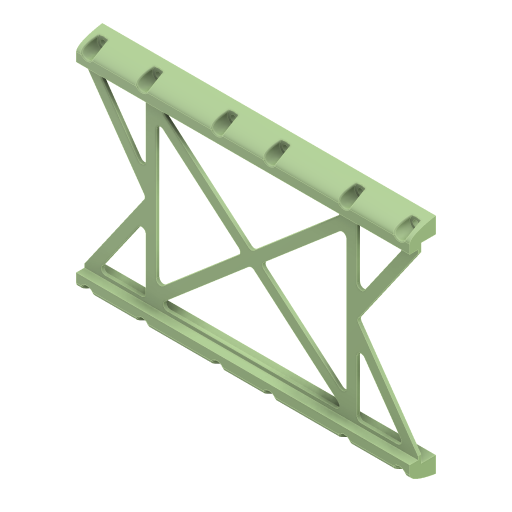
# Autodesk Inventor part: BodyStructure Centre Bottom
Saved by Autodesk Inventor 2023 (Build 270158000, 158)
## iProperties
Created: 2019-11-07
Part Number: BodyStructure Centre Bottom
Material: solidworks materials|ABS
Document SubType Name: Modeling
Designer: Jochen
Density: 1.02 g/cm^3
Appearance: 151,157,178
Sending System: SolidWorks 2017
Last Author: Felix
Last Saved: 2021-02-23
Author: Jochen
Autodesk Inventor part; units mm, degrees
note: some values were not read from the file. Chosen so that the rebuilt part matches the saved one: second side of "Extrusion1".
ref_plane "YZ Plane" through (0, 0, 0) normal (1, 0, 0) x (0, 1, 0)
ref_plane "XZ Plane" through (0, 0, 0) normal (0, 1, 0) x (-1, 0, 0)
ref_plane "Work Plane1" through (0, 0, 30) normal (0, 0, 1) x (1, 0, 0)
sketch "Sketch1" plane through (0, 0, 30) normal (0, 0, 1) x (1, 0, 0)
  line L0 (-80, -55) -> (80, -55)
  line L1 (80, 55) -> (-80, 55)
  line L2 (80, 42) -> (80, 42)
  line L3 (0, -77) -> (0, 77) construction
  line L4 (-112, 0) -> (112, 0) construction
  line L5 (-50.649, -42) -> (-50.649, -8.7287)
  line L6 (-45.649, 35.4185) -> (-45.649, -35.4185)
  line L7 (-50.649, -8.7287) -> (-73.9001, -42)
  line L8 (-80, -42) -> (-50.649, 0)
  line L9 (50.649, -8.7287) -> (73.9001, -42)
  line L10 (50.649, -42) -> (50.649, -8.7287)
  line L11 (45.649, 35.4185) -> (45.649, -35.4185)
  line L12 (80, -42) -> (50.649, 0)
  line L13 (50.649, 8.7287) -> (73.9001, 42)
  line L14 (80, 42) -> (50.649, 0)
  line L15 (50.649, 0) -> (50.649, 0)
  line L16 (50.649, 8.7287) -> (50.649, 42)
  line L17 (-50.649, 0) -> (-50.649, 0)
  line L18 (-80, 42) -> (-50.649, 0)
  line L19 (-50.649, 8.7287) -> (-73.9001, 42)
  line L20 (-80, 42) -> (-80, 42)
  line L21 (-50.649, 8.7287) -> (-50.649, 42)
  line L22 (73.9001, 42) -> (50.649, 42)
  line L23 (-73.9001, 42) -> (-50.649, 42)
  line L24 (-45.649, 42) -> (45.649, 42)
  line L25 (-80, -42) -> (-80, -42)
  line L26 (-50.649, -42) -> (-73.9001, -42)
  line L27 (45.649, -42) -> (-45.649, -42)
  line L28 (80, -42) -> (80, -42)
  line L29 (73.9001, -42) -> (50.649, -42)
  line L30 (80, -55) -> (80, -42)
  line L31 (80, 42) -> (80, 55)
  line L32 (-80, 55) -> (-80, 42)
  line L33 (-80, -42) -> (-80, -55)
  line L34 (-48.149, 55) -> (-48.149, -55) construction
  line L35 (-45.649, 42) -> (0, 2.9266)
  line L36 (0, 2.9266) -> (45.649, 42)
  line L37 (45.649, 35.4185) -> (4.2699, 0)
  line L38 (45.649, -35.4185) -> (4.2699, 0)
  line L39 (0, -2.9266) -> (45.649, -42)
  line L40 (-4.2699, 0) -> (-45.649, 35.4185)
  line L41 (-4.2699, 0) -> (-45.649, -35.4185)
  line L42 (0, -2.9266) -> (-45.649, -42)
  point P0 (0, 0)
  point P1 (-2.5, 42)
  point P2 (2.5, 42)
  point P3 (2.5, -42)
  point P4 (-2.5, -42)
  point P5 (50.649, 0)
  point P6 (-50.649, 0)
  dimension "d2" = 5
  dimension "d3" = 0
  dimension "d4" = 160
  dimension "d5" = 13
  dimension "d7" = 110
  dimension "d101" = 5
  dimension "d107" = 5
  constraints: 82 end point, 17 parallel, 15 collinear, 15 perpendicular, 11 point on line, 9 horizontal, 2 vertical, 19 other
  measures "d2" distance between parallel lines of L6 L5
  measures "d3" distance of L8.start L25.end
  measures "d4" distance of L0.start L0.end
  measures "d5" distance of L25.end L0.start
  measures "d7" distance between parallel lines of L1 L0
  measures "d101" distance between parallel lines of L8 L7
  measures "d107" distance between parallel lines of L42 L41
extrude "Extrusion1" add sketch "Sketch1" along normal blind 15.5
fillet "Fillet1" radius 2 22 edges at (-50.649, -42, 37.75) (-50.649, -8.7287, 37.75) (-73.9001, -42, 37.75) (-73.9001, 42, 37.75) (-50.649, 42, 37.75) (-50.649, 8.7287, 37.75) (50.649, -8.7287, 37.75) (50.649, -42, 37.75) (50.649, 42, 37.75) (50.649, 8.7287, 37.75) (73.9001, 42, 37.75) (73.9001, -42, 37.75) (-45.649, 35.4185, 37.75) (0, -2.9266, 37.75) (4.2699, 0, 37.75) (0, 2.9266, 37.75) (-4.2699, 0, 37.75) (-45.649, -35.4185, 37.75) (45.649, -35.4185, 37.75) (45.649, 35.4185, 37.75) (50.649, 0, 37.75) (-50.649, 0, 37.75)
fillet "Fillet1" radius 2 4 edges at (-45.649, 42, 37.75) (-45.649, -42, 37.75) (45.649, -42, 37.75) (45.649, 42, 37.75)
sketch "Sketch3" plane through (0, 0, 0) normal (1, 0, 0) x (0, 1, 0)
  line L0 (0, -9.1414) -> (0, 54.8485) construction
  line L1 (-78.4953, 0) -> (85.9718, 0) construction
  line L2 (-42, 45.5) -> (-55, 45.5) construction
  line L3 (-55, 45.5) -> (-42, 45.5) construction
  line L4 (-42, 45.5) -> (-1.1456, 45.5) construction
  line L5 (1.1456, 45.5) -> (42, 45.5) construction
  line L6 (42, 45.5) -> (55, 45.5) construction
  line L7 (55, 45.5) -> (42, 45.5) construction
  line L8 (42, 45.5) -> (1.1456, 45.5) construction
  line L9 (-1.1456, 45.5) -> (-42, 45.5) construction
  line L10 (13.9365, 45.5) -> (38.8544, 45.5) construction
  line L11 (42, 45.5) -> (38.8544, 45.5) construction
  line L12 (40, 45.5) -> (42, 45.5) construction
  line L13 (40, 45.5) -> (15.0821, 45.5) construction
  line L14 (13.9365, 45.5) -> (15.0821, 45.5) construction
  line L15 (15.0821, 45.5) -> (40, 45.5) construction
  line L16 (42, 45.5) -> (40, 45.5) construction
  line L17 (38.8544, 45.5) -> (42, 45.5) construction
  line L18 (38.8544, 45.5) -> (13.9365, 45.5) construction
  line L19 (15.0821, 45.5) -> (13.9365, 45.5) construction
  line L20 (-13.9365, 45.5) -> (-38.8544, 45.5) construction
  line L21 (-40, 45.5) -> (-42, 45.5) construction
  line L22 (-40, 45.5) -> (-15.0821, 45.5) construction
  line L23 (-13.9365, 45.5) -> (-15.0821, 45.5) construction
  line L24 (-38.8544, 45.5) -> (-42, 45.5) construction
  line L25 (-38.8544, 45.5) -> (-13.9365, 45.5) construction
  line L26 (-15.0821, 45.5) -> (-13.9365, 45.5) construction
  line L27 (-15.0821, 45.5) -> (-40, 45.5) construction
  line L28 (-42, 45.5) -> (-40, 45.5) construction
  line L29 (-42, 30) -> (-55, 30) construction
  line L30 (-1.1456, 30) -> (-42, 30) construction
  line L31 (42, 30) -> (1.1456, 30) construction
  line L32 (55, 30) -> (42, 30) construction
  line L33 (42, 30) -> (55, 30) construction
  line L34 (1.1456, 30) -> (42, 30) construction
  line L35 (-42, 30) -> (-1.1456, 30) construction
  line L36 (-55, 30) -> (-42, 30) construction
  line L37 (15.0821, 30) -> (13.9365, 30) construction
  line L38 (40, 30) -> (15.0821, 30) construction
  line L39 (42, 30) -> (40, 30) construction
  line L40 (38.8544, 30) -> (42, 30) construction
  line L41 (13.9365, 30) -> (38.8544, 30) construction
  line L42 (13.9365, 30) -> (15.0821, 30) construction
  line L43 (38.8544, 30) -> (13.9365, 30) construction
  line L44 (42, 30) -> (38.8544, 30) construction
  line L45 (40, 30) -> (42, 30) construction
  line L46 (15.0821, 30) -> (40, 30) construction
  line L47 (-15.0821, 30) -> (-13.9365, 30) construction
  line L48 (-40, 30) -> (-15.0821, 30) construction
  line L49 (-42, 30) -> (-40, 30) construction
  line L50 (-13.9365, 30) -> (-38.8544, 30) construction
  line L51 (-40, 30) -> (-42, 30) construction
  line L52 (-15.0821, 30) -> (-40, 30) construction
  line L53 (-13.9365, 30) -> (-15.0821, 30) construction
  line L54 (-38.8544, 30) -> (-13.9365, 30) construction
  line L55 (-42, 30) -> (-38.8544, 30) construction
  line L56 (55, 30) -> (55, 45.5) construction
  line L57 (55, 30) -> (55, 45.5) construction
  line L58 (-55, 30) -> (-55, 45.5) construction
  line L59 (-55, 30) -> (-55, 45.5) construction
  line L60 (-37, 30) -> (-37, 45.5) construction
  line L61 (-37, 30) -> (-37, 45.5) construction
  line L62 (-55, 30) -> (-55, 45.5)
  line L63 (-47.5, 45.5) -> (-45, 45.5)
  line L64 (-43.75, 41.5) -> (43.75, 41.5)
  line L65 (55, 45.5) -> (55, 30)
  line L66 (55, 30) -> (-55, 30)
  line L67 (-46.25, 45.5) -> (-46.25, 30) construction
  line L68 (-38.8544, 30) -> (-42, 30) projected
  line L69 (-42, 45.5) -> (-38.8544, 45.5) projected
  line L70 (42, 45.5) -> (42, 30) projected
  line L71 (42, 30) -> (42, 45.5) projected
  line L72 (1.1456, 30) -> (-1.1456, 30) projected
  line L73 (-1.1456, 30) -> (1.1456, 30) projected
  line L74 (1.1456, 45.5) -> (-1.1456, 45.5) projected
  line L75 (-1.1456, 45.5) -> (1.1456, 45.5) projected
  line L76 (-43.75, 41.5) -> (-43.75, 45.5)
  line L77 (-43.75, 45.5) -> (-45, 45.5)
  line L78 (-55, 45.5) -> (-42, 45.5) projected
  line L79 (-47.5, 45.5) -> (-55, 45.5)
  line L80 (-55, 30) -> (-55, 45.5) projected
  line L81 (42, 45.5) -> (55, 45.5) projected
  line L82 (43.75, 41.5) -> (43.75, 45.5)
  line L83 (55, 45.5) -> (43.75, 45.5)
  point P0 (0, 0)
  point P1 (-55, 39.9819)
  point P2 (62.4765, 45.5)
  dimension "d114" = 4
  dimension "d115" = 87.5
  constraints: 25 end point, 8 point on line, 4 perpendicular, 3 collinear, 2 horizontal, 2 vertical, 1 midpoint, 1 parallel, 6 other
  measures "d114" distance of L64.start L76.end
  measures "d115" distance between parallel lines of L76 L82
extrude "Extrusion3" cut sketch "Sketch3" along normal through all both and the other way through all contours L62 L78 L63 L77 L76 L64 L70 L66 | L70 L64 L82 L81 L65 L66 keep common part
sketch "Sketch12" plane through (80, -55, 30) normal (1, 0, 0) x (0, 0, -1)
  line L0 (0, 13) -> (0, 0) projected
  line L1 (0, 0) -> (-15.5, 0) projected
  line L2 (-15.5, 110) -> (0, 110) projected
  line L3 (0, 110) -> (0, 97) projected
  line L4 (-11.5, 13) -> (0, 13) projected
  line L5 (0, 97) -> (-11.5, 97) projected
  line L6 (-11.5, 97) -> (-11.5, 98.75) projected
  line L7 (-11.5, 98.75) -> (-15.5, 98.75) projected
  line L8 (-15.5, 98.75) -> (-15.5, 110) projected
  line L9 (-15.5, 0) -> (-15.5, 11.25) projected
  line L10 (-15.5, 11.25) -> (-11.5, 11.25) projected
  line L11 (-11.5, 11.25) -> (-11.5, 13) projected
  point P0 (30, 55)
  point P1 (-11.5, 11.4559)
  point P2 (-11.5, 98.5441)
sketch "Sketch15" plane through (0, 0, 0) normal (0, 1, 0) x (-1, 0, 0)
  line L0 (-51.089, 41.5) -> (-45.649, 41.5) construction
  line L1 (-45.649, 41.5) -> (-45.649, 30) construction
  line L2 (-45.649, 30) -> (-51.089, 30) construction
  line L3 (-51.089, 30) -> (-51.089, 41.5) construction
  line L4 (-5.3456, 41.5) -> (5.3456, 41.5) construction
  line L5 (5.3456, 41.5) -> (5.3456, 30) construction
  line L6 (5.3456, 30) -> (-5.3456, 30) construction
  line L7 (-5.3456, 30) -> (-5.3456, 41.5) construction
  line L8 (45.649, 41.5) -> (51.089, 41.5) construction
  line L9 (51.089, 41.5) -> (51.089, 30) construction
  line L10 (51.089, 30) -> (45.649, 30) construction
  line L11 (45.649, 30) -> (45.649, 41.5) construction
  line L12 (-27.5, 45.5) -> (-8.5, 45.5)
  line L13 (-8.5, 44.5) -> (-8.5, 30)
  line L14 (-8.5, 30) -> (-28.5, 30)
  line L15 (-28.5, 30) -> (-28.5, 44.5)
  line L16 (-8.5, 30) -> (8.5, 30)
  line L17 (8.5, 30) -> (8.5, 44.5)
  line L18 (7.5, 45.5) -> (-7.5, 45.5)
  line L19 (-8.5, 45.5) -> (-8.5, 30)
  line L20 (8.5, 30) -> (28.5, 30)
  line L21 (28.5, 30) -> (28.5, 44.5)
  line L22 (27.5, 45.5) -> (8.5, 45.5)
  line L23 (8.5, 45.5) -> (8.5, 30)
  line L24 (80, 45.5) -> (-80, 45.5) construction
  line L25 (-42.3485, 30) -> (-6.0451, 30) construction
  arc A0 (-27.5, 45.5) -> (-28.5, 44.5) centre (-27.5, 44.5) ccw
  arc A1 (28.5, 44.5) -> (27.5, 45.5) centre (27.5, 44.5) ccw
  arc A2 (8.5, 44.5) -> (7.5, 45.5) centre (7.5, 44.5) ccw
  arc A3 (-7.5, 45.5) -> (-8.5, 44.5) centre (-7.5, 44.5) ccw
  line L26 (-8.5, 45.5) -> (-7.5, 45.5)
  line L27 (7.5, 45.5) -> (8.5, 45.5)
  line L28 (28.5, 36.2) -> (-28.5, 36.2)
  point P0 (0, 0)
  point P1 (-28.5, 45.5)
  point P2 (28.5, 45.5)
  point P3 (28.5, 37.25)
  point P4 (-8.5, 36.2)
  point P5 (8.5, 36.2)
  dimension "d123" = 37
  dimension "d124" = 37
  dimension "d125" = 51.5
  dimension "d126" = 51.5
  dimension "d131" = 1
  dimension "d133" = 9.3
  constraints: 30 end point, 16 point on line, 10 tangent, 9 point on circle, 6 parallel, 4 centre point, 4 horizontal, 3 equal radius, 3 perpendicular, 2 collinear, 1 midpoint
  measures "d123" distance between parallel lines of L17 L15
  measures "d124" distance from line of point (28.5, 37.25) L13
  measures "d125" distance from line of L15 L24.end
  measures "d126" horizontal distance of L24.start L20.end
  measures "d131" radius of A0
  measures "d133" distance between parallel lines of L28 L24
sketch "Sketch16" plane through (0, 0, 0) normal (1, 0, 0) x (0, 1, 0)
  line L0 (-80.8624, 0) -> (80.8624, 0) construction
  line L1 (-80.8624, 0) -> (80.8624, 0) construction
  line L2 (0, -29.7721) -> (0, 58.7721) construction
  line L3 (-48, 45.5) -> (-48, -16.5) construction
  line L4 (55, 45.5) -> (43.75, 45.5) construction
  line L5 (48, 45.5) -> (48, -16.5) construction
  line L6 (-43.75, 45.5) -> (-55, 45.5) construction
  ellipse E0 centre (-48, 14.5) end of major axis (-48, 45.5) minor radius 7 (-48, 45.5) -> (-55, 14.5) ccw
  line L7 (-55, 30) -> (-55, 45.5) projected
  line L8 (-55, 30) -> (-55, 14.5) construction
  line L9 (-48, 45.5) -> (-55, 45.5)
  line L10 (-55, 45.5) -> (-55, 14.5)
  ellipse E1 centre (48, 14.5) end of major axis (48, 45.5) minor radius 7 (48, -16.5) -> (55, 14.5) ccw construction
  line L11 (48, 45.5) -> (55, 45.5)
  line L12 (55, 45.5) -> (55, 14.5)
  ellipse E2 centre (-48, 14.5) end of major axis (-48, 45.5) minor radius 7 (-55, 14.5) -> (-48, -16.5) ccw construction
  ellipse E3 centre (48, 14.5) end of major axis (48, 45.5) minor radius 7 (55, 14.5) -> (48, 45.5) ccw
  line L13 (55, 14.5) -> (-55, 14.5) construction
  point P0 (0, 0)
  dimension "d138" = 62
  dimension "d139" = 7
  constraints: 16 end point, 8 vertical, 2 collinear, 2 midpoint, 2 point on line, 1 horizontal, 1 parallel, 17 other
  measures "d138" distance of L3.end L3.start
  measures "d139" distance from line of L3 L6.end
extrude "Extrusion16" cut sketch "Sketch16" along normal through all both and the other way through all
sketch "Sketch5" plane through (0, 0, 0) normal (0, 1, 0) x (-1, 0, 0)
  line L0 (112, 0) -> (-112, 0) construction
  line L1 (0, -9.1414) -> (0, 54.8485) construction
  line L2 (80, 41.5) -> (80, 45.5) construction
  line L3 (-80, 30) -> (-80, 45.5) construction
  line L4 (-80, 30) -> (80, 30) construction
  line L5 (80, 30) -> (80, 45.5) construction
  line L6 (80, 39.5) -> (80, 41.5) construction
  line L7 (-80, 41.5) -> (-80, 39.5) construction
  line L8 (-52, 34.5) -> (-52, 33)
  line L9 (-52, 33) -> (-45, 33)
  line L10 (-45, 33) -> (-45, 40)
  line L11 (-45, 40) -> (-16, 40)
  line L12 (-16, 40) -> (-16, 33)
  line L13 (-16, 33) -> (-9, 33)
  line L14 (-9, 33) -> (-9, 40)
  line L15 (-9, 40) -> (9, 40)
  line L16 (9, 40) -> (9, 33)
  line L17 (9, 33) -> (16, 33)
  line L18 (16, 33) -> (16, 40)
  line L19 (16, 40) -> (45, 40)
  line L20 (45, 40) -> (45, 33)
  line L21 (45, 33) -> (52, 33)
  line L22 (52, 33) -> (52, 34.5)
  line L23 (80, 34.5) -> (80, 45.5)
  line L24 (80, 30) -> (-80, 30) construction
  line L25 (-80, 45.5) -> (-80, 34.5)
  line L26 (80, 41.5) -> (-80, 41.5)
  line L27 (52, 34.5) -> (80, 34.5)
  line L28 (-80, 34.5) -> (-52, 34.5)
  line L29 (52, 40) -> (45, 40) construction
  line L30 (80, 45.5) -> (-80, 45.5) projected
  line L31 (-80, 45.5) -> (80, 45.5)
  line L32 (-80, 45.5) -> (80, 45.5) projected
  line L33 (-52.649, 30) -> (-52.649, 41.5) projected
  line L34 (53, 34.5) -> (53, 33)
  line L35 (53, 33) -> (52, 33)
  line L36 (-53, 34.5) -> (-53, 33)
  line L37 (-53, 33) -> (-52, 33)
  line L38 (-45, 33) -> (45, 33)
  line L39 (45.649, 41.5) -> (45.649, 30) projected
  line L40 (53, 33) -> (80, 33)
  line L41 (-53, 33) -> (-80, 33)
  line L42 (-80, 34.5) -> (-80, 33)
  line L43 (-80, 30) -> (-80, 41.5) projected
  line L44 (80, 34.5) -> (80, 33)
  line L45 (80, 30) -> (80, 41.5) projected
  point P0 (0, 0)
  point P1 (61.4737, 40)
  point P2 (56.7369, 40)
  point P3 (48.5, 33)
  point P4 (-52.649, 34.5)
  dimension "d47" = 7
  dimension "d48" = 9
  dimension "d51" = 11
  dimension "d96" = 7
  dimension "d102" = 48.5
  dimension "d118" = 12.5
  dimension "d145" = 27
  dimension "d146" = 27
  constraints: 62 end point, 16 point on line, 15 perpendicular, 6 collinear, 3 vertical, 1 horizontal, 1 midpoint, 1 parallel, 2 other
  measures "d47" distance between parallel lines of L22 L20
  measures "d48" distance between parallel lines of L1 L16
  measures "d51" distance from line of L2.end L27
  measures "d96" distance between parallel lines of L21 L29
  measures "d102" distance from line of L1 point (48.5, 33)
  measures "d118" distance between parallel lines of L30 L13
  measures "d145" distance between parallel lines of L5 L34
  measures "d146" distance between parallel lines of L3 L36
extrude "Extrusion5" cut sketch "Sketch5" along normal through all both and the other way through all keep common part
sketch "Sketch6" plane through (0, 0, 0) normal (1, 0, 0) x (0, 1, 0)
  line L0 (0, -9.1414) -> (0, 54.8485) construction
  line L1 (-77, 0) -> (77, 0) construction
  line L2 (-38.535, 41.5) -> (-36.9915, 41.5) construction
  line L3 (-45.875, 40) -> (-45.875, 25)
  line L4 (-45.875, 25) -> (45.875, 25)
  line L5 (45.875, 25) -> (45.875, 40)
  line L6 (-45.875, 40) -> (45.875, 40)
  line L7 (42, 40) -> (51.9805, 40) projected
  line L8 (-43.75, 45.5) -> (-48, 45.5) construction
  line L9 (45.875, 25) -> (53.125, 25)
  line L10 (53.125, 25) -> (53.125, 40)
  line L11 (45.875, 40) -> (53.125, 40)
  line L12 (-45.875, 40) -> (-53.125, 40)
  line L13 (-53.125, 40) -> (-53.125, 25)
  line L14 (-53.125, 25) -> (-45.875, 25)
  line L15 (55, 33) -> (55, 40) projected
  line L16 (55, 33) -> (55, 25)
  line L17 (55, 25) -> (53.125, 25)
  line L18 (55, 33) -> (55, 40)
  line L19 (55, 40) -> (53.125, 40)
  line L20 (-53.125, 25) -> (-55, 25)
  line L21 (-55, 25) -> (-55, 40)
  line L22 (-55, 40) -> (-53.125, 40)
  point P0 (0, 0)
  point P1 (-45.875, 32.5)
  point P2 (54.9365, 40)
  point P3 (-45, 45.5)
  point P4 (-47.5, 45.5)
  point P5 (-45.875, 45.5)
  point P6 (55, 39.5)
  point P7 (-55, 33)
  point P8 (55, 39.5)
  point P9 (54.9365, 40)
  point P10 (-54.9365, 40)
  point P11 (-54.9161, 45.5)
  point P12 (-50, 45.5)
  point P13 (54.9791, 40)
  point P14 (-42, 45.5)
  point P15 (-55, 45.5)
  dimension "d75" = 1.5
  dimension "d104" = 15
  dimension "d106" = 7.25
  constraints: 37 end point, 6 perpendicular, 6 point on line, 4 collinear, 2 horizontal, 2 vertical, 1 midpoint, 1 parallel, 3 other
  measures "d75" distance between parallel lines of L6 L2
  measures "d104" distance from line of L6 L3.end
  measures "d106" distance between parallel lines of L5 L10
extrude "Extrusion6" cut sketch "Sketch6" along normal mid plane 160 contours L6 L5 L4 L3
sketch "Sketch9" plane through (45, -54.9365, 40) normal (0, 0, -1) x (-1, 0, 0)
  line L0 (-35, 100.8115) -> (-35, 106.917) projected
  line L1 (-35, 2.956) -> (-35, 9.0615) projected
  line L2 (125, 106.917) -> (125, 100.8115) projected
  line L3 (125, 9.0615) -> (125, 2.956) projected
  circle A0 centre (-30, 104.9365) radius 1.5
  circle A1 centre (32.5, 104.9365) radius 1.5
  circle A2 centre (-3.5, 104.9365) radius 1.5
  circle A3 centre (57.5, 104.9365) radius 1.5
  circle A4 centre (93.5, 104.9365) radius 1.5
  circle A5 centre (120, 104.9365) radius 1.5
  circle A6 centre (120, 4.9365) radius 1.5
  circle A7 centre (93.5, 4.9365) radius 1.5
  circle A8 centre (57.5, 4.9365) radius 1.5
  circle A9 centre (-3.5, 4.9365) radius 1.5
  circle A10 centre (32.5, 4.9365) radius 1.5
  circle A11 centre (-30, 4.9365) radius 1.5
  line L4 (-30, 104.9365) -> (120, 104.9365) construction
  line L5 (120, 104.9365) -> (120, 4.9365) construction
  line L6 (120, 4.9365) -> (-30, 4.9365) construction
  line L7 (-30, 4.9365) -> (-30, 104.9365) construction
  line L8 (157, 54.9365) -> (-67, 54.9365) construction
  line L9 (45, -22.0635) -> (45, 131.9365) construction
  line L10 (32.5, 104.9365) -> (32.5, 4.9365) construction
  line L11 (-3.5, 4.9365) -> (-3.5, 104.9365) construction
  line L12 (93.5, 104.9365) -> (93.5, 4.9365) construction
  line L13 (57.5, 104.9365) -> (57.5, 4.9365) construction
  circle A12 centre (-30, 4.9365) radius 2.9
  circle A13 centre (-3.5, 4.9365) radius 2.9
  circle A14 centre (32.5, 4.9365) radius 2.9
  circle A15 centre (57.5, 4.9365) radius 2.9
  circle A16 centre (93.5, 4.9365) radius 2.9
  circle A17 centre (120, 4.9365) radius 2.9
  circle A18 centre (120, 104.9365) radius 2.9
  circle A19 centre (93.5, 104.9365) radius 2.9
  circle A20 centre (57.5, 104.9365) radius 2.9
  circle A21 centre (32.5, 104.9365) radius 2.9
  circle A22 centre (-3.5, 104.9365) radius 2.9
  circle A23 centre (-30, 104.9365) radius 2.9
  line L14 (125, 108.4365) -> (-35, 108.4365)
  line L15 (-35, 1.4365) -> (125, 1.4365)
  line L16 (-35, 9.0615) -> (125, 9.0615) projected
  line L17 (125, 100.8115) -> (-35, 100.8115) projected
  line L18 (97.7, 1.4365) -> (97.7, -0.0635)
  line L19 (97.7, 108.4365) -> (97.7, 109.9365)
  line L20 (125, -0.0635) -> (-35, -0.0635) projected
  line L21 (-7.7, -0.0635) -> (-7.7, 1.4365)
  line L22 (-7.7, 108.4365) -> (-7.7, 109.9365)
  line L23 (125, 109.9365) -> (-35, 109.9365) projected
  line L24 (125, 2.956) -> (-35, 2.956) projected
  line L25 (-35, 106.917) -> (125, 106.917) projected
  arc A24 (-25.0624, 96.9365) -> (-26.7018, 93.7909) centre (-25.0624, 94.9365) ccw projected
  line L26 (-26.7018, 93.7909) -> (-9.2884, 68.873) projected
  arc A25 (-9.2884, 68.873) -> (-5.649, 70.0186) centre (-7.649, 70.0186) ccw projected
  line L27 (-5.649, 70.0186) -> (-5.649, 94.9365) projected
  arc A26 (-5.649, 94.9365) -> (-7.649, 96.9365) centre (-7.649, 94.9365) ccw projected
  line L28 (-7.649, 96.9365) -> (-25.0624, 96.9365) projected
  line L29 (99.2884, 68.873) -> (116.7018, 93.7909) projected
  arc A27 (116.7018, 93.7909) -> (115.0624, 96.9365) centre (115.0624, 94.9365) ccw projected
  line L30 (115.0624, 96.9365) -> (97.649, 96.9365) projected
  arc A28 (97.649, 96.9365) -> (95.649, 94.9365) centre (97.649, 94.9365) ccw projected
  line L31 (95.649, 94.9365) -> (95.649, 70.0186) projected
  arc A29 (95.649, 70.0186) -> (99.2884, 68.873) centre (97.649, 70.0186) ccw projected
  arc A30 (99.2884, 41) -> (95.649, 39.8543) centre (97.649, 39.8543) ccw projected
  line L32 (95.649, 39.8543) -> (95.649, 14.9365) projected
  arc A31 (95.649, 14.9365) -> (97.649, 12.9365) centre (97.649, 14.9365) ccw projected
  line L33 (97.649, 12.9365) -> (115.0624, 12.9365) projected
  arc A32 (115.0624, 12.9365) -> (116.7018, 16.0821) centre (115.0624, 14.9365) ccw projected
  line L34 (116.7018, 16.0821) -> (99.2884, 41) projected
  line L35 (86.5373, 16.4559) -> (46.3005, 50.8966) projected
  arc A33 (46.3005, 50.8966) -> (43.6995, 50.8966) centre (45, 49.3772) ccw projected
  line L36 (43.6995, 50.8966) -> (3.4627, 16.4559) projected
  arc A34 (3.4627, 16.4559) -> (4.7632, 12.9365) centre (4.7632, 14.9365) ccw projected
  line L37 (4.7632, 12.9365) -> (85.2368, 12.9365) projected
  arc A35 (85.2368, 12.9365) -> (86.5373, 16.4559) centre (85.2368, 14.9365) ccw projected
  line L38 (3.4627, 93.4171) -> (43.6995, 58.9763) projected
  arc A36 (43.6995, 58.9763) -> (46.3005, 58.9763) centre (45, 60.4957) ccw projected
  line L39 (46.3005, 58.9763) -> (86.5373, 93.4171) projected
  arc A37 (86.5373, 93.4171) -> (85.2368, 96.9365) centre (85.2368, 94.9365) ccw projected
  line L40 (85.2368, 96.9365) -> (4.7632, 96.9365) projected
  arc A38 (4.7632, 96.9365) -> (3.4627, 93.4171) centre (4.7632, 94.9365) ccw projected
  line L41 (2.6515, 22.3431) -> (38.9549, 53.4171) projected
  arc A39 (38.9549, 53.4171) -> (38.9549, 56.4559) centre (37.6544, 54.9365) ccw projected
  line L42 (38.9549, 56.4559) -> (2.6515, 87.5299) projected
  arc A40 (2.6515, 87.5299) -> (-0.649, 86.0105) centre (1.351, 86.0105) ccw projected
  line L43 (-0.649, 86.0105) -> (-0.649, 23.8625) projected
  arc A41 (-0.649, 23.8625) -> (2.6515, 22.3431) centre (1.351, 23.8625) ccw projected
  line L44 (90.649, 23.8625) -> (90.649, 86.0105) projected
  arc A42 (90.649, 86.0105) -> (87.3485, 87.5299) centre (88.649, 86.0105) ccw projected
  line L45 (87.3485, 87.5299) -> (51.0451, 56.4559) projected
  arc A43 (51.0451, 56.4559) -> (51.0451, 53.4171) centre (52.3456, 54.9365) ccw projected
  line L46 (51.0451, 53.4171) -> (87.3485, 22.3431) projected
  arc A44 (87.3485, 22.3431) -> (90.649, 23.8625) centre (88.649, 23.8625) ccw projected
  line L47 (-5.649, 14.9365) -> (-5.649, 39.8543) projected
  arc A45 (-5.649, 39.8543) -> (-9.2884, 41) centre (-7.649, 39.8543) ccw projected
  line L48 (-9.2884, 41) -> (-26.7018, 16.0821) projected
  arc A46 (-26.7018, 16.0821) -> (-25.0624, 12.9365) centre (-25.0624, 14.9365) ccw projected
  line L49 (-25.0624, 12.9365) -> (-7.649, 12.9365) projected
  arc A47 (-7.649, 12.9365) -> (-5.649, 14.9365) centre (-7.649, 14.9365) ccw projected
  line L50 (125, 96.9365) -> (96.4496, 56.0821) projected
  arc A48 (96.4496, 56.0821) -> (96.4496, 53.7909) centre (98.089, 54.9365) ccw projected
  line L51 (96.4496, 53.7909) -> (125, 12.9365) projected
  line L52 (125, 12.9365) -> (125, 9.0615) projected
  line L53 (125, 100.8115) -> (125, 96.9365) projected
  line L54 (-35, 9.0615) -> (-35, 12.9365) projected
  line L55 (-35, 12.9365) -> (-6.4496, 53.7909) projected
  arc A49 (-6.4496, 53.7909) -> (-6.4496, 56.0821) centre (-8.089, 54.9365) ccw projected
  line L56 (-6.4496, 56.0821) -> (-35, 96.9365) projected
  line L57 (-35, 96.9365) -> (-35, 100.8115) projected
  point P0 (45, 54.9365)
  point P1 (42.5, 12.9365)
  point P2 (-6, 80.6486)
  point P3 (-6, 19.2244)
  point P4 (-6, 14.9365)
  point P5 (47.5, 86.9365)
  point P6 (42.5, 76.9365)
  point P7 (42.5, 22.9365)
  point P8 (47.5, 76.9365)
  point P9 (47.5, 22.9365)
  point P10 (-6, 36.0374)
  point P11 (98.4175, 46.8521)
  point P12 (45, 52.0098)
  point P13 (45, 57.8631)
  point P14 (-5.649, 54.9365)
  point P15 (95.649, 54.9365)
  point P16 (0, 109.9365)
  point P17 (36, -0.0635)
  point P18 (29, -0.0635)
  point P19 (0, -0.0635)
  point P20 (1, 109.9365)
  point P21 (28, 109.9365)
  point P22 (37, 109.9365)
  point P23 (53, 109.9365)
  point P24 (62, 109.9365)
  point P25 (89, 109.9365)
  point P26 (98, 109.9365)
  point P27 (89, -0.0635)
  point P28 (62, -0.0635)
  point P29 (53, -0.0635)
  point P30 (37, -0.0635)
  point P31 (28, -0.0635)
  point P32 (1, -0.0635)
  point P33 (-8, -0.0635)
  point P34 (0, 101.8115)
  point P35 (90, 101.8115)
  point P36 (90, 8.0615)
  point P37 (0, 8.0615)
  point P38 (36.5, -0.0635)
  point P39 (16.5, 109.9365)
  point P40 (16.5, -0.0635)
  dimension "d61" = 3
  dimension "d63" = 100
  dimension "d64" = 75
  dimension "d65" = 48.5
  dimension "d66" = 12.5
  dimension "d69" = 5.8
  constraints: 28 end point, 24 centre point, 22 equal radius, 17 point on line, 15 coincident, 4 perpendicular, 3 parallel, 2 collinear, 2 vertical, 1 horizontal, 8 other
  measures "d61" diameter of A0
  measures "d63" distance of L6.end L4.start
  measures "d64" distance from line of A11.centre L9
  measures "d65" distance from line of L11.start L9
  measures "d66" distance from line of L10.end L9
  measures "d69" diameter of A12
extrude "Extrusion8" cut sketch "Sketch9" along normal through all both and the other way through all contours A0 | A1 | A2 | A3 | A4 | A5 | A6 | A7 | A8 | A9 | A10 | A11
extrude "Extrusion9" cut sketch "Sketch9" along normal blind 8 from surface at -5.5 contours L25 A23 | A23 L25 | L25 A18 | A18 L25 | L25 A22 | A22 L25 | L25 A19 | A19 L25 | L25 A21 | A21 L25 | L25 A20 | A20 L25 | L24 A12 | A12 L24 | L24 A17 | A17 L24 | L24 A13 | A13 L24 | L24 A16 | A16 L24 | L24 A14 | A14 L24 | L24 A15 | A15 L24 | A0 | A1 | A2 | A3 | A4 | A5 | A6 | A7 | A8 | A9 | A10 | A11
sketch "Sketch10" plane through (0, 0, 0) normal (1, 0, 0) x (0, 1, 0)
  line L0 (-77, 0) -> (77, 0) construction
  line L1 (0, -9.1414) -> (0, 54.8485) construction
  line L2 (-43.5, 40) -> (43.5, 40)
  line L3 (43.5, 40) -> (43.5, 34.5)
  line L4 (43.5, 34.5) -> (-43.5, 34.5)
  line L5 (-43.5, 34.5) -> (-43.5, 40)
  line L6 (29.1214, 34.5) -> (55, 34.5) construction
  point P0 (0, 0)
  dimension "d105" = 87
  constraints: 8 end point, 2 parallel, 1 horizontal, 1 perpendicular, 1 point on line, 1 other
  measures "d105" distance of L3.end L4.end
extrude "Extrusion10" cut sketch "Sketch10" along normal through all both and the other way through all
extrude "Extrusion17" add sketch "Sketch9" along normal blind 3 from surface at 2.5 contours L25 A23 | A23 L25 | L25 A18 | A18 L25 | L25 A22 | A22 L25 | L25 A19 | A19 L25 | L25 A21 | A21 L25 | L25 A20 | A20 L25 | L24 A12 | A12 L24 | L24 A17 | A17 L24 | L24 A13 | A13 L24 | L24 A16 | A16 L24 | L24 A14 | A14 L24 | L24 A15 | A15 L24
fillet "Fillet6" radius 0.5 12 edges at (75, 47.1, 45.5) (48.5, 47.1, 45.5) (12.5, 47.1, 45.5) (-12.5, 47.1, 45.5) (-48.5, 47.1, 45.5) (-75, 47.1, 45.5) (-75, -47.1, 45.5) (-48.5, -47.1, 45.5) (-12.5, -47.1, 45.5) (12.5, -47.1, 45.5) (48.5, -47.1, 45.5) (75, -47.1, 45.5)
equation "\"d2\" = d1"
equation "\"d1\" = 5"
body "Solid1"
body "Solid2"
